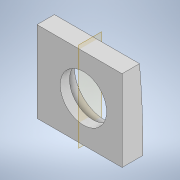
# Autodesk Inventor part: irrigation02
Saved by Autodesk Inventor 2021.1 (Build 251245000, 245)
## iProperties
Created: 2020-08-29
Part Number: irrigation02
Material: Generic
Document SubType Name: Modeling
Designer: robst
Density: 1 g/cm^3
Appearance: Default
Author: robst
Autodesk Inventor part; units mm, degrees
ref_plane "XZ Plane" through (0, 0, 0) normal (0, 1, 0) x (-1, 0, 0)
sketch "Sketch1" plane through (0, 0, 0) normal (1, 0, 0) x (0, 1, 0)
  line L0 (0, 0) -> (0, 12.7)
  line L1 (0, 0) -> (-101.6, 0) construction
  arc A0 (-101.6, 0) -> (0, 0) centre (-50.8, 556.4861) ccw
  line L2 (-50.8, -2.3139) -> (-50.8, 0) construction
  line L3 (0, 12.7) -> (101.6, 12.7) construction
  arc A1 (0, 12.7) -> (101.6, 12.7) centre (50.8, 569.1861) ccw
  line L4 (0, 12.7) -> (-53.34, 12.7)
  line L5 (-53.34, 12.7) -> (-53.34, -2.3081)
  dimension "d0" = 12.7
  dimension "d1" = 101.6
  dimension "d5" = 558.8
  dimension "d6" = 101.6
  dimension "d7" = 558.8
  dimension "d8" = 53.34
  constraints: 12 end point, 6 point on circle, 3 horizontal, 2 centre point, 1 midpoint, 1 perpendicular, 1 vertical
  measures "d0" distance of L0.start L0.end
  measures "d1" distance of L0.start L1.end
  measures "d5" radius of A0
  measures "d6" distance of L0.end L3.end
  measures "d7" radius of A1
  measures "d8" distance of L0.end L4.end
extrude "Extrusion1" add sketch "Sketch1" along normal mid plane 55.88
sketch "Sketch2" plane through (-27.94, -53.34, 12.7) normal (0, 0, 1) x (1, 0, 0)
  line L0 (0, 0) -> (55.88, 0) construction
  circle A0 centre (30.48, 26.67) radius 15.24
  line L1 (0, 53.34) -> (55.88, 53.34)
  line L2 (0, 0) -> (0, 53.34) projected
  point P0 (27.94, 53.34)
  dimension "d11" = 30.48
  dimension "d12" = 26.67
  dimension "d22" = 30.48
  constraints: 2 end point, 1 centre point
  measures "d11" diameter of A0
  measures "d12" distance from line of A0.centre L1
  measures "d22" distance from line of A0.centre L2
extrude "Extrusion2" cut sketch "Sketch2" against normal through all
ref_plane "Work Plane2" through (0, -50.8, -2.3139) normal (0, 0, 1) x (1, 0, 0)
sketch "Sketch3" plane through (0, -50.8, -2.3139) normal (0, 0, 1) x (1, 0, 0)
  spline S0 degree 2 poles (17.78, 24.13) (17.78, 50.5265) (-5.08, 37.3282) (-27.94, 24.13) (-5.08, 10.9318) (17.78, -2.2665) (17.78, 24.13) knots 0 0 0 0.333333 0.333333 0.666667 0.666667 1 1 1 weights 1 0.5 1 0.5 1 0.5 1 projected
  circle A0 centre (2.54, 24.13) radius 15.24 projected
  circle A1 centre (2.54, 24.13) radius 19.05
  point P0 (0, 50.8)
  dimension "d15" = 3.81
  constraints: 1 centre point, 1 coincident, 1 vertical alignment, 1 other
extrude "Extrusion3" cut sketch "Sketch3" along normal blind 7.62
sketch "Sketch4" plane through (0, -50.8, -2.3139) normal (0, 0, 1) x (1, 0, 0)
  line L0 (27.94, -2.54) -> (27.94, 50.8) construction
  line L1 (27.94, 46.355) -> (-26.8216, 46.355)
  line L2 (-27.94, 50.8) -> (27.94, 50.8) construction
  line L3 (23.8128, 44.45) -> (24.2945, 44.45)
  line L4 (24.2945, 44.45) -> (24.2945, 47.309)
  line L5 (24.2945, 47.309) -> (23.8128, 47.309)
  line L6 (23.8128, 47.309) -> (23.8128, 44.45)
  line L7 (23.7789, 47.7845) -> (24.3254, 47.7845)
  line L8 (24.3254, 47.7845) -> (24.3254, 48.2847)
  line L9 (24.3254, 48.2847) -> (23.7789, 48.2847)
  line L10 (23.7789, 48.2847) -> (23.7789, 47.7845)
  line L11 (21.5898, 46.7934) -> (21.6145, 46.7934)
  spline S0 degree 2 poles (21.6145, 46.7934) (21.6701, 46.8089) (21.7905, 46.815) (21.8739, 46.815) knots 0 0 0 1 2 2 2
  spline S1 degree 2 poles (21.8739, 46.815) (22.0684, 46.815) (22.4512, 46.6452) (22.6241, 46.4785) knots 0 0 0 1 2 2 2
  line L12 (22.6241, 46.4785) -> (22.6241, 44.45)
  line L13 (22.6241, 44.45) -> (23.1058, 44.45)
  line L14 (23.1058, 44.45) -> (23.1058, 47.309)
  line L15 (23.1058, 47.309) -> (22.6241, 47.309)
  line L16 (22.6241, 47.309) -> (22.6241, 46.883)
  spline S2 degree 2 poles (22.6241, 46.883) (22.3617, 47.1176) (21.9696, 47.309) (21.7843, 47.309) knots 0 0 0 1 2 2 2
  spline S3 degree 2 poles (21.7843, 47.309) (21.7102, 47.309) (21.6361, 47.3029) (21.5898, 47.2936) knots 0 0 0 1 2 2 2
  line L17 (21.5898, 47.2936) -> (21.5898, 46.7934)
  line L18 (19.7003, 46.7934) -> (19.725, 46.7934)
  spline S4 degree 2 poles (19.725, 46.7934) (19.7805, 46.8089) (19.9009, 46.815) (19.9843, 46.815) knots 0 0 0 1 2 2 2
  spline S5 degree 2 poles (19.9843, 46.815) (20.1788, 46.815) (20.5617, 46.6452) (20.7346, 46.4785) knots 0 0 0 1 2 2 2
  line L19 (20.7346, 46.4785) -> (20.7346, 44.45)
  line L20 (20.7346, 44.45) -> (21.2162, 44.45)
  line L21 (21.2162, 44.45) -> (21.2162, 47.309)
  line L22 (21.2162, 47.309) -> (20.7346, 47.309)
  line L23 (20.7346, 47.309) -> (20.7346, 46.883)
  spline S6 degree 2 poles (20.7346, 46.883) (20.4721, 47.1176) (20.08, 47.309) (19.8948, 47.309) knots 0 0 0 1 2 2 2
  spline S7 degree 2 poles (19.8948, 47.309) (19.8207, 47.309) (19.7466, 47.3029) (19.7003, 47.2936) knots 0 0 0 1 2 2 2
  line L24 (19.7003, 47.2936) -> (19.7003, 46.7934)
  spline S8 degree 2 poles (17.0265, 46.355) (17.0265, 45.3299) (17.6224, 44.3697) (18.2429, 44.3697) knots 0 0 0 1 2 2 2
  spline S9 degree 2 poles (18.2429, 44.3697) (18.8728, 44.3697) (19.4625, 45.3485) (19.4625, 46.3519) knots 0 0 0 1 2 2 2
  spline S10 degree 2 poles (19.4625, 46.3519) (19.4625, 47.3831) (18.8666, 48.3372) (18.2429, 48.3372) knots 0 0 0 1 2 2 2
  spline S11 degree 2 poles (18.2429, 48.3372) (17.6162, 48.3372) (17.0265, 47.3492) (17.0265, 46.355) knots 0 0 0 1 2 2 2
  spline S12 degree 2 poles (17.681, 45.1941) (17.6069, 45.3824) (17.5452, 45.9629) (17.5452, 46.355) knots 0 0 0 1 2 2 2
  spline S13 degree 2 poles (17.5452, 46.355) (17.5452, 46.7471) (17.6069, 47.3245) (17.6841, 47.519) knots 0 0 0 1 2 2 2
  spline S14 degree 2 poles (17.6841, 47.519) (17.7613, 47.7135) (18.0299, 47.9142) (18.2429, 47.9142) knots 0 0 0 1 2 2 2
  spline S15 degree 2 poles (18.2429, 47.9142) (18.456, 47.9142) (18.7308, 47.7135) (18.8111, 47.5128) knots 0 0 0 1 2 2 2
  spline S16 degree 2 poles (18.8111, 47.5128) (18.8882, 47.3183) (18.9438, 46.7255) (18.9438, 46.3519) knots 0 0 0 1 2 2 2
  spline S17 degree 2 poles (18.9438, 46.3519) (18.9438, 45.9505) (18.8944, 45.4133) (18.8141, 45.2034) knots 0 0 0 1 2 2 2
  spline S18 degree 2 poles (18.8141, 45.2034) (18.74, 45.0058) (18.4652, 44.7927) (18.2429, 44.7927) knots 0 0 0 1 2 2 2
  spline S19 degree 2 poles (18.2429, 44.7927) (18.033, 44.7927) (17.7582, 44.9934) (17.681, 45.1941) knots 0 0 0 1 2 2 2
  line L25 (14.189, 44.45) -> (16.5386, 44.45)
  line L26 (16.5386, 44.45) -> (16.5386, 44.9903)
  spline S20 degree 2 poles (16.5386, 44.9903) (16.2855, 45.2281) (15.8347, 45.6696) (15.6186, 45.9073) knots 0 0 0 1 2 2 2
  spline S21 degree 2 poles (15.6186, 45.9073) (15.1832, 46.3859) (14.8652, 46.9602) (14.8652, 47.2658) knots 0 0 0 1 2 2 2
  spline S22 degree 2 poles (14.8652, 47.2658) (14.8652, 47.4264) (14.964, 47.6672) (15.0535, 47.7444) knots 0 0 0 1 2 2 2
  spline S23 degree 2 poles (15.0535, 47.7444) (15.1431, 47.8216) (15.3777, 47.8988) (15.5198, 47.8988) knots 0 0 0 1 2 2 2
  spline S24 degree 2 poles (15.5198, 47.8988) (15.6556, 47.8988) (15.9335, 47.8308) (16.0601, 47.7783) knots 0 0 0 1 2 2 2
  spline S25 degree 2 poles (16.0601, 47.7783) (16.1681, 47.7351) (16.3688, 47.6116) (16.4306, 47.5684) knots 0 0 0 1 2 2 2
  line L27 (16.4306, 47.5684) -> (16.4584, 47.5684)
  line L28 (16.4584, 47.5684) -> (16.4584, 48.1118)
  spline S26 degree 2 poles (16.4584, 48.1118) (16.3009, 48.189) (15.7359, 48.3403) (15.4827, 48.3403) knots 0 0 0 1 2 2 2
  spline S27 degree 2 poles (15.4827, 48.3403) (14.9486, 48.3403) (14.3465, 47.7753) (14.3465, 47.2936) knots 0 0 0 1 2 2 2
  spline S28 degree 2 poles (14.3465, 47.2936) (14.3465, 47.0682) (14.4515, 46.6915) (14.5441, 46.531) knots 0 0 0 1 2 2 2
  spline S29 degree 2 poles (14.5441, 46.531) (14.6367, 46.3643) (14.9053, 46.037) (15.0535, 45.8795) knots 0 0 0 1 2 2 2
  spline S30 degree 2 poles (15.0535, 45.8795) (15.2944, 45.6171) (15.8841, 45.0552) (16.0601, 44.8915) knots 0 0 0 1 2 2 2
  line L29 (16.0601, 44.8915) -> (14.189, 44.8915)
  line L30 (14.189, 44.8915) -> (14.189, 44.45)
  line L31 (11.0459, 44.45) -> (11.0459, 47.8092)
  line L32 (11.0459, 47.8092) -> (12.3242, 47.8092)
  line L33 (12.3242, 47.8092) -> (12.3242, 48.26)
  line L34 (12.3242, 48.26) -> (9.2614, 48.26)
  line L35 (9.2614, 48.26) -> (9.2614, 47.8092)
  line L36 (9.2614, 47.8092) -> (10.5396, 47.8092)
  line L37 (10.5396, 47.8092) -> (10.5396, 44.45)
  line L38 (10.5396, 44.45) -> (11.0459, 44.45)
  spline S31 degree 2 poles (6.1769, 47.8247) (5.9608, 47.5715) (5.72, 46.8305) (5.72, 46.355) knots 0 0 0 1 2 2 2
  spline S32 degree 2 poles (5.72, 46.355) (5.72, 45.8919) (5.9546, 45.1416) (6.1769, 44.8884) knots 0 0 0 1 2 2 2
  spline S33 degree 2 poles (6.1769, 44.8884) (6.4116, 44.6229) (7.0322, 44.3697) (7.4058, 44.3697) knots 0 0 0 1 2 2 2
  spline S34 degree 2 poles (7.4058, 44.3697) (7.7917, 44.3697) (8.4092, 44.6322) (8.6346, 44.8884) knots 0 0 0 1 2 2 2
  spline S35 degree 2 poles (8.6346, 44.8884) (8.8538, 45.1416) (9.0884, 45.8857) (9.0884, 46.355) knots 0 0 0 1 2 2 2
  spline S36 degree 2 poles (9.0884, 46.355) (9.0884, 46.8336) (8.8507, 47.5622) (8.6315, 47.8247) knots 0 0 0 1 2 2 2
  spline S37 degree 2 poles (8.6315, 47.8247) (8.4092, 48.0778) (7.7886, 48.3403) (7.4058, 48.3403) knots 0 0 0 1 2 2 2
  spline S38 degree 2 poles (7.4058, 48.3403) (7.0167, 48.3403) (6.393, 48.0686) (6.1769, 47.8247) knots 0 0 0 1 2 2 2
  spline S39 degree 2 poles (6.2479, 46.355) (6.2479, 46.7317) (6.4116, 47.3152) (6.5598, 47.5066) knots 0 0 0 1 2 2 2
  spline S40 degree 2 poles (6.5598, 47.5066) (6.7111, 47.7042) (7.1371, 47.9018) (7.4027, 47.9018) knots 0 0 0 1 2 2 2
  spline S41 degree 2 poles (7.4027, 47.9018) (7.6775, 47.9018) (8.0912, 47.7104) (8.2486, 47.5066) knots 0 0 0 1 2 2 2
  spline S42 degree 2 poles (8.2486, 47.5066) (8.3999, 47.3121) (8.5605, 46.7255) (8.5605, 46.355) knots 0 0 0 1 2 2 2
  spline S43 degree 2 poles (8.5605, 46.355) (8.5605, 45.6047) (7.9306, 44.8082) (7.4027, 44.8082) knots 0 0 0 1 2 2 2
  spline S44 degree 2 poles (7.4027, 44.8082) (6.8747, 44.8082) (6.2479, 45.6047) (6.2479, 46.355) knots 0 0 0 1 2 2 2
  spline S45 degree 2 poles (2.7559, 47.1114) (2.7559, 46.8644) (2.9319, 46.4198) (3.0894, 46.2655) knots 0 0 0 1 2 2 2
  spline S46 degree 2 poles (3.0894, 46.2655) (3.287, 46.0709) (3.8211, 45.8703) (4.2287, 45.8703) knots 0 0 0 1 2 2 2
  line L39 (4.2287, 45.8703) -> (4.6579, 45.8703)
  line L40 (4.6579, 45.8703) -> (4.6579, 44.45)
  line L41 (4.6579, 44.45) -> (5.1642, 44.45)
  line L42 (5.1642, 44.45) -> (5.1642, 48.26)
  line L43 (5.1642, 48.26) -> (4.2071, 48.26)
  spline S47 degree 2 poles (4.2071, 48.26) (3.8675, 48.26) (3.392, 48.1488) (3.2098, 48.0223) knots 0 0 0 1 2 2 2
  spline S48 degree 2 poles (3.2098, 48.0223) (2.9968, 47.8771) (2.7559, 47.4295) (2.7559, 47.1114) knots 0 0 0 1 2 2 2
  spline S49 degree 2 poles (3.2839, 47.096) (3.2839, 47.2936) (3.4198, 47.5838) (3.5587, 47.6765) knots 0 0 0 1 2 2 2
  spline S50 degree 2 poles (3.5587, 47.6765) (3.6791, 47.7567) (4.0002, 47.8216) (4.238, 47.8216) knots 0 0 0 1 2 2 2
  line L44 (4.238, 47.8216) -> (4.6579, 47.8216)
  line L45 (4.6579, 47.8216) -> (4.6579, 46.3025)
  line L46 (4.6579, 46.3025) -> (4.3121, 46.3025)
  spline S51 degree 2 poles (4.3121, 46.3025) (4.0033, 46.3025) (3.6235, 46.4013) (3.5, 46.531) knots 0 0 0 1 2 2 2
  spline S52 degree 2 poles (3.5, 46.531) (3.3858, 46.6452) (3.2839, 46.9138) (3.2839, 47.096) knots 0 0 0 1 2 2 2
  line L47 (0.7985, 48.4298) -> (2.2897, 43.6225)
  line L48 (2.2897, 43.6225) -> (2.722, 43.6225)
  line L49 (2.722, 43.6225) -> (1.2369, 48.4298)
  line L50 (1.2369, 48.4298) -> (0.7985, 48.4298)
  spline S53 degree 2 poles (-2.3138, 45.6202) (-2.3138, 45.3361) (-2.0976, 44.9008) (-1.9186, 44.7588) knots 0 0 0 1 2 2 2
  spline S54 degree 2 poles (-1.9186, 44.7588) (-1.7024, 44.592) (-1.2115, 44.45) (-0.8225, 44.45) knots 0 0 0 1 2 2 2
  line L51 (-0.8225, 44.45) -> (0.2705, 44.45)
  line L52 (0.2705, 44.45) -> (0.2705, 48.26)
  line L53 (0.2705, 48.26) -> (-0.7391, 48.26)
  spline S55 degree 2 poles (-0.7391, 48.26) (-1.1467, 48.26) (-1.5542, 48.2075) (-1.7395, 48.1056) knots 0 0 0 1 2 2 2
  spline S56 degree 2 poles (-1.7395, 48.1056) (-1.9463, 47.9976) (-2.1347, 47.6425) (-2.1347, 47.4017) knots 0 0 0 1 2 2 2
  spline S57 degree 2 poles (-2.1347, 47.4017) (-2.1347, 47.1331) (-1.8506, 46.707) (-1.6005, 46.5866) knots 0 0 0 1 2 2 2
  line L54 (-1.6005, 46.5866) -> (-1.6005, 46.568)
  spline S58 degree 2 poles (-1.6005, 46.568) (-1.9402, 46.4754) (-2.3138, 45.9845) (-2.3138, 45.6202) knots 0 0 0 1 2 2 2
  spline S59 degree 2 poles (-1.7858, 45.5986) (-1.7858, 45.8147) (-1.6623, 46.0926) (-1.477, 46.1914) knots 0 0 0 1 2 2 2
  spline S60 degree 2 poles (-1.477, 46.1914) (-1.3566, 46.2531) (-1.0726, 46.2902) (-0.8101, 46.2902) knots 0 0 0 1 2 2 2
  line L55 (-0.8101, 46.2902) -> (-0.2359, 46.2902)
  line L56 (-0.2359, 46.2902) -> (-0.2359, 44.8823)
  line L57 (-0.2359, 44.8823) -> (-0.6465, 44.8823)
  spline S61 degree 2 poles (-0.6465, 44.8823) (-0.98, 44.8823) (-1.3628, 44.944) (-1.511, 45.0428) knots 0 0 0 1 2 2 2
  spline S62 degree 2 poles (-1.511, 45.0428) (-1.653, 45.1447) (-1.7858, 45.3979) (-1.7858, 45.5986) knots 0 0 0 1 2 2 2
  spline S63 degree 2 poles (-1.6067, 47.3307) (-1.6067, 47.4665) (-1.5141, 47.6703) (-1.4122, 47.7289) knots 0 0 0 1 2 2 2
  spline S64 degree 2 poles (-1.4122, 47.7289) (-1.2887, 47.7969) (-0.9892, 47.8277) (-0.7206, 47.8277) knots 0 0 0 1 2 2 2
  line L58 (-0.7206, 47.8277) -> (-0.2359, 47.8277)
  line L59 (-0.2359, 47.8277) -> (-0.2359, 46.7132)
  line L60 (-0.2359, 46.7132) -> (-0.8101, 46.7132)
  spline S65 degree 2 poles (-0.8101, 46.7132) (-1.0479, 46.7132) (-1.2733, 46.7626) (-1.3937, 46.8397) knots 0 0 0 1 2 2 2
  spline S66 degree 2 poles (-1.3937, 46.8397) (-1.511, 46.9138) (-1.6067, 47.1516) (-1.6067, 47.3307) knots 0 0 0 1 2 2 2
  line L61 (-2.4064, 44.45) -> (-3.6908, 48.26)
  line L62 (-3.6908, 48.26) -> (-4.3145, 48.26)
  line L63 (-4.3145, 48.26) -> (-5.5989, 44.45)
  line L64 (-5.5989, 44.45) -> (-5.0647, 44.45)
  line L65 (-5.0647, 44.45) -> (-4.7189, 45.5152)
  line L66 (-4.7189, 45.5152) -> (-3.2647, 45.5152)
  line L67 (-3.2647, 45.5152) -> (-2.9189, 44.45)
  line L68 (-2.9189, 44.45) -> (-2.4064, 44.45)
  line L69 (-4.58, 45.9474) -> (-3.9903, 47.7413)
  line L70 (-3.9903, 47.7413) -> (-3.4037, 45.9474)
  line L71 (-3.4037, 45.9474) -> (-4.58, 45.9474)
  spline S67 degree 2 poles (-7.4977, 44.3821) (-7.1272, 44.3821) (-6.5004, 44.6322) (-6.272, 44.8823) knots 0 0 0 1 2 2 2
  spline S68 degree 2 poles (-6.272, 44.8823) (-6.0435, 45.1293) (-5.7934, 45.8703) (-5.7934, 46.3519) knots 0 0 0 1 2 2 2
  spline S69 degree 2 poles (-5.7934, 46.3519) (-5.7934, 46.8305) (-6.0373, 47.5406) (-6.2689, 47.803) knots 0 0 0 1 2 2 2
  spline S70 degree 2 poles (-6.2689, 47.803) (-6.4974, 48.0593) (-7.121, 48.3279) (-7.507, 48.3279) knots 0 0 0 1 2 2 2
  spline S71 degree 2 poles (-7.507, 48.3279) (-7.6984, 48.3279) (-8.0349, 48.2724) (-8.177, 48.2291) knots 0 0 0 1 2 2 2
  spline S72 degree 2 poles (-8.177, 48.2291) (-8.3005, 48.189) (-8.5567, 48.0747) (-8.6833, 48.0068) knots 0 0 0 1 2 2 2
  line L72 (-8.6833, 48.0068) -> (-8.6833, 47.3955)
  line L73 (-8.6833, 47.3955) -> (-8.6432, 47.3955)
  spline S73 degree 2 poles (-8.6432, 47.3955) (-8.5753, 47.4572) (-8.3653, 47.6301) (-8.214, 47.7135) knots 0 0 0 1 2 2 2
  spline S74 degree 2 poles (-8.214, 47.7135) (-8.0689, 47.7938) (-7.7262, 47.8957) (-7.5039, 47.8957) knots 0 0 0 1 2 2 2
  spline S75 degree 2 poles (-7.5039, 47.8957) (-7.26, 47.8957) (-6.8246, 47.695) (-6.661, 47.5036) knots 0 0 0 1 2 2 2
  spline S76 degree 2 poles (-6.661, 47.5036) (-6.5004, 47.309) (-6.3214, 46.7193) (-6.3214, 46.3519) knots 0 0 0 1 2 2 2
  spline S77 degree 2 poles (-6.3214, 46.3519) (-6.3214, 45.9598) (-6.5097, 45.3948) (-6.6733, 45.2003) knots 0 0 0 1 2 2 2
  spline S78 degree 2 poles (-6.6733, 45.2003) (-6.8339, 45.0119) (-7.2631, 44.8205) (-7.5039, 44.8205) knots 0 0 0 1 2 2 2
  spline S79 degree 2 poles (-7.5039, 44.8205) (-7.7231, 44.8205) (-8.0967, 44.9286) (-8.2418, 45.0088) knots 0 0 0 1 2 2 2
  spline S80 degree 2 poles (-8.2418, 45.0088) (-8.3807, 45.0891) (-8.5876, 45.2558) (-8.6463, 45.3145) knots 0 0 0 1 2 2 2
  line L74 (-8.6463, 45.3145) -> (-8.6833, 45.3145)
  line L75 (-8.6833, 45.3145) -> (-8.6833, 44.7094)
  spline S81 degree 2 poles (-8.6833, 44.7094) (-8.5567, 44.6507) (-8.3344, 44.5426) (-8.177, 44.4932) knots 0 0 0 1 2 2 2
  spline S82 degree 2 poles (-8.177, 44.4932) (-8.0102, 44.4376) (-7.7262, 44.3821) (-7.4977, 44.3821) knots 0 0 0 1 2 2 2
  line L76 (-11.9345, 44.45) -> (-11.2768, 44.45)
  line L77 (-11.2768, 44.45) -> (-9.8844, 46.2222)
  line L78 (-9.8844, 46.2222) -> (-9.6621, 45.9721)
  line L79 (-9.6621, 45.9721) -> (-9.6621, 44.45)
  line L80 (-9.6621, 44.45) -> (-9.1557, 44.45)
  line L81 (-9.1557, 44.45) -> (-9.1557, 48.26)
  line L82 (-9.1557, 48.26) -> (-9.6621, 48.26)
  line L83 (-9.6621, 48.26) -> (-9.6621, 46.5094)
  line L84 (-9.6621, 46.5094) -> (-11.2243, 48.26)
  line L85 (-11.2243, 48.26) -> (-11.8419, 48.26)
  line L86 (-11.8419, 48.26) -> (-10.2641, 46.5588)
  line L87 (-10.2641, 46.5588) -> (-11.9345, 44.45)
  spline S83 degree 2 poles (-16.2817, 47.1114) (-16.2817, 46.8644) (-16.1057, 46.4198) (-15.9483, 46.2655) knots 0 0 0 1 2 2 2
  spline S84 degree 2 poles (-15.9483, 46.2655) (-15.7507, 46.0709) (-15.2165, 45.8703) (-14.809, 45.8703) knots 0 0 0 1 2 2 2
  line L88 (-14.809, 45.8703) -> (-14.3798, 45.8703)
  line L89 (-14.3798, 45.8703) -> (-14.3798, 44.45)
  line L90 (-14.3798, 44.45) -> (-13.8734, 44.45)
  line L91 (-13.8734, 44.45) -> (-13.8734, 48.26)
  line L92 (-13.8734, 48.26) -> (-14.8306, 48.26)
  spline S85 degree 2 poles (-14.8306, 48.26) (-15.1702, 48.26) (-15.6457, 48.1488) (-15.8278, 48.0223) knots 0 0 0 1 2 2 2
  spline S86 degree 2 poles (-15.8278, 48.0223) (-16.0409, 47.8771) (-16.2817, 47.4295) (-16.2817, 47.1114) knots 0 0 0 1 2 2 2
  spline S87 degree 2 poles (-15.7537, 47.096) (-15.7537, 47.2936) (-15.6179, 47.5838) (-15.479, 47.6765) knots 0 0 0 1 2 2 2
  spline S88 degree 2 poles (-15.479, 47.6765) (-15.3585, 47.7567) (-15.0374, 47.8216) (-14.7997, 47.8216) knots 0 0 0 1 2 2 2
  line L93 (-14.7997, 47.8216) -> (-14.3798, 47.8216)
  line L94 (-14.3798, 47.8216) -> (-14.3798, 46.3025)
  line L95 (-14.3798, 46.3025) -> (-14.7256, 46.3025)
  spline S89 degree 2 poles (-14.7256, 46.3025) (-15.0343, 46.3025) (-15.4141, 46.4013) (-15.5376, 46.531) knots 0 0 0 1 2 2 2
  spline S90 degree 2 poles (-15.5376, 46.531) (-15.6519, 46.6452) (-15.7537, 46.9138) (-15.7537, 47.096) knots 0 0 0 1 2 2 2
  line L96 (-19.5267, 48.26) -> (-18.2145, 44.45)
  line L97 (-18.2145, 44.45) -> (-17.668, 44.45)
  line L98 (-17.668, 44.45) -> (-16.3558, 48.26)
  line L99 (-16.3558, 48.26) -> (-16.8992, 48.26)
  line L100 (-16.8992, 48.26) -> (-17.9551, 45.0953)
  line L101 (-17.9551, 45.0953) -> (-19.0111, 48.26)
  line L102 (-19.0111, 48.26) -> (-19.5267, 48.26)
  spline S91 degree 2 poles (-22.1974, 46.355) (-22.1974, 45.3299) (-21.6015, 44.3697) (-20.9809, 44.3697) knots 0 0 0 1 2 2 2
  spline S92 degree 2 poles (-20.9809, 44.3697) (-20.3511, 44.3697) (-19.7613, 45.3485) (-19.7613, 46.3519) knots 0 0 0 1 2 2 2
  spline S93 degree 2 poles (-19.7613, 46.3519) (-19.7613, 47.3831) (-20.3572, 48.3372) (-20.9809, 48.3372) knots 0 0 0 1 2 2 2
  spline S94 degree 2 poles (-20.9809, 48.3372) (-21.6077, 48.3372) (-22.1974, 47.3492) (-22.1974, 46.355) knots 0 0 0 1 2 2 2
  spline S95 degree 2 poles (-21.5428, 45.1941) (-21.6169, 45.3824) (-21.6787, 45.9629) (-21.6787, 46.355) knots 0 0 0 1 2 2 2
  spline S96 degree 2 poles (-21.6787, 46.355) (-21.6787, 46.7471) (-21.6169, 47.3245) (-21.5398, 47.519) knots 0 0 0 1 2 2 2
  spline S97 degree 2 poles (-21.5398, 47.519) (-21.4626, 47.7135) (-21.194, 47.9142) (-20.9809, 47.9142) knots 0 0 0 1 2 2 2
  spline S98 degree 2 poles (-20.9809, 47.9142) (-20.7679, 47.9142) (-20.4931, 47.7135) (-20.4128, 47.5128) knots 0 0 0 1 2 2 2
  spline S99 degree 2 poles (-20.4128, 47.5128) (-20.3356, 47.3183) (-20.28, 46.7255) (-20.28, 46.3519) knots 0 0 0 1 2 2 2
  spline S100 degree 2 poles (-20.28, 46.3519) (-20.28, 45.9505) (-20.3294, 45.4133) (-20.4097, 45.2034) knots 0 0 0 1 2 2 2
  spline S101 degree 2 poles (-20.4097, 45.2034) (-20.4838, 45.0058) (-20.7586, 44.7927) (-20.9809, 44.7927) knots 0 0 0 1 2 2 2
  spline S102 degree 2 poles (-20.9809, 44.7927) (-21.1909, 44.7927) (-21.4657, 44.9934) (-21.5428, 45.1941) knots 0 0 0 1 2 2 2
  spline S103 degree 2 poles (-24.9947, 45.6603) (-24.9947, 45.3855) (-24.8187, 44.9162) (-24.6581, 44.7433) knots 0 0 0 1 2 2 2
  spline S104 degree 2 poles (-24.6581, 44.7433) (-24.4976, 44.5704) (-24.019, 44.3697) (-23.7226, 44.3697) knots 0 0 0 1 2 2 2
  spline S105 degree 2 poles (-23.7226, 44.3697) (-23.4509, 44.3697) (-22.9199, 44.4901) (-22.7254, 44.5859) knots 0 0 0 1 2 2 2
  line L103 (-22.7254, 44.5859) -> (-22.7254, 45.1262)
  line L104 (-22.7254, 45.1262) -> (-22.7624, 45.1262)
  spline S106 degree 2 poles (-22.7624, 45.1262) (-22.8211, 45.0829) (-23.0403, 44.9718) (-23.1731, 44.9224) knots 0 0 0 1 2 2 2
  spline S107 degree 2 poles (-23.1731, 44.9224) (-23.3243, 44.8699) (-23.5744, 44.8112) (-23.7319, 44.8112) knots 0 0 0 1 2 2 2
  spline S108 degree 2 poles (-23.7319, 44.8112) (-23.8863, 44.8112) (-24.1765, 44.9224) (-24.2815, 45.0428) knots 0 0 0 1 2 2 2
  spline S109 degree 2 poles (-24.2815, 45.0428) (-24.3772, 45.157) (-24.476, 45.4596) (-24.476, 45.6634) knots 0 0 0 1 2 2 2
  spline S110 degree 2 poles (-24.476, 45.6634) (-24.476, 45.8672) (-24.3648, 46.1265) (-24.2599, 46.213) knots 0 0 0 1 2 2 2
  spline S111 degree 2 poles (-24.2599, 46.213) (-24.1518, 46.3087) (-23.8307, 46.389) (-23.6362, 46.389) knots 0 0 0 1 2 2 2
  spline S112 degree 2 poles (-23.6362, 46.389) (-23.4262, 46.389) (-23.0094, 46.3241) (-22.8828, 46.2963) knots 0 0 0 1 2 2 2
  line L105 (-22.8828, 46.2963) -> (-22.8828, 48.26)
  line L106 (-22.8828, 48.26) -> (-24.9731, 48.26)
  line L107 (-24.9731, 48.26) -> (-24.9731, 47.8123)
  line L108 (-24.9731, 47.8123) -> (-23.3737, 47.8123)
  line L109 (-23.3737, 47.8123) -> (-23.3737, 46.7965)
  spline S113 degree 2 poles (-23.3737, 46.7965) (-23.4664, 46.8089) (-23.6454, 46.8181) (-23.7195, 46.8181) knots 0 0 0 1 2 2 2
  spline S114 degree 2 poles (-23.7195, 46.8181) (-24.0129, 46.8181) (-24.4173, 46.7224) (-24.6026, 46.5804) knots 0 0 0 1 2 2 2
  spline S115 degree 2 poles (-24.6026, 46.5804) (-24.7909, 46.4384) (-24.9947, 46.0061) (-24.9947, 45.6603) knots 0 0 0 1 2 2 2
  point P0 (0, 50.8)
  dimension "d18" = 4.445
  constraints: 2 end point, 2 horizontal, 1 point on line
  measures "d18" distance between parallel lines of L1 L2
emboss "Emboss1" sketch "Sketch4" operation cut depth 1.27 direction (0, 0, -1) wrap yes faces at (0.2009, -50.7671, -2.3139) contours S12 S19 S18 S17 S16 L1 S10 S9 S8 | L1 S11 S10 S16 S15 S14 S13 | S35 S34 S33 S32 L1 S44 S43 | L1 S42 S41 S40 S39 S31 S38 S37 S36 | S95 S102 S101 S100 S99 L1 S93 S92 S91 | L1 S94 S93 S99 S98 S97 S96 | L4 L3 L6 L1 | L1 L6 L5 L4 | L14 L13 L12 L1 | L1 L12 S1 S0 L11 L17 S3 S2 L16 L15 L14 | L21 L20 L19 L1 | L1 L19 S5 S4 L18 L24 S7 S6 L23 L22 L21 | S21 S20 L26 L25 L30 L29 S30 S29 L1 | L1 S29 S28 S27 S26 L28 L27 S25 S24 S23 S22 S21 | L31 L38 L37 L1 | L1 L37 L36 L35 L34 L33 L32 L31 | L42 L41 L40 L39 S46 S45 L1 S51 L46 L45 | L1 L45 L44 S50 S49 S52 S51 S45 S48 S47 L43 L42 | L49 L48 L47 L1 | L1 L47 L50 L49 | L52 L51 S54 S53 S58 L1 | L1 S58 L54 S57 S56 S55 L53 L52 | L61 L68 L67 L66 L65 L64 L63 L1 L69 L71 L70 | L1 L70 L69 L63 L62 L61 | S69 S68 S67 S82 S81 L75 L74 S80 S79 S78 S77 S76 L1 | L1 S76 S75 S74 S73 L73 L72 S72 S71 S70 S69 | L81 L80 L79 L78 L77 L76 L87 L1 | L1 L87 L86 L85 L84 L83 L82 L81 | L91 L90 L89 L88 S84 S83 L1 S89 L95 L94 | L1 L94 L93 S88 S87 S90 S89 S83 S86 S85 L92 L91 | L98 L97 L96 L1 L101 L100 | L1 L100 L99 L98 | L1 L96 L102 L101 | L105 S112 L1 | L1 S112 S111 S115 S114 S113 L109 L108 L107 L106 L105 | S111 S110 S109 S108 S107 S106 L104 L103 S105 S104 S103 S115 L1 | L10 L9 L8 L7
sketch "Sketch5" plane through (0, 0, 0) normal (1, 0, 0) x (0, 1, 0)
  line L0 (0, 0) -> (0, 12.7) projected
  line L1 (0, 12.7) -> (-53.34, 12.7) projected
  line L2 (-53.34, 12.7) -> (-53.34, -2.3081) projected
  line L3 (0, 12.7) -> (-53.34, 12.7)
  line L4 (-53.34, 12.7) -> (-53.34, 11.43)
  line L5 (-53.34, 11.43) -> (0, 11.43)
  line L6 (0, 11.43) -> (0, 12.7)
  point P0 (0, 11.43)
  dimension "d23" = 1.27
  constraints: 8 end point, 2 parallel, 1 horizontal, 1 perpendicular, 1 point on line
  measures "d23" distance between parallel lines of L1 L5
extrude "Extrusion4" cut sketch "Sketch5" against normal through all both and the other way through all
equation "\"d0\" = sidingDepth"
equation "\"d1\" = sidingHeight"
equation "\"d5\" = radiusOfCurvature"
equation "\"d6\" = sidingHeight"
equation "\"d7\" = radiusOfCurvature"
equation "\"d8\" = partHeight"
equation "\"d9\" = partWidth"
equation "\"d11\" = pipeDiameter"
equation "\"d12\" = pipeCenter"
equation "\"d15\" = clearanceRingForBackHole"
equation "\"d16\" = clearanceDepth"
equation "\"d18\" = textLine"
equation "\"d19\" = textDepth"
equation "\"sidingHeight\" = 101.6"
equation "\"sidingDepth\" = 12.7"
equation "\"radiusOfCurvature\" = 558.8"
equation "\"pipeDiameter\" = 30.48"
equation "\"partWidth\" = 55.88"
equation "\"partHeight\" = 53.34"
equation "\"pipeCenter\" = 26.67"
equation "\"clearanceRingForBackHole\" = 3.81"
equation "\"clearanceDepth\" = 7.62"
equation "\"textLine\" = 4.445"
equation "\"textDepth\" = 1.27"
body "Solid1"
